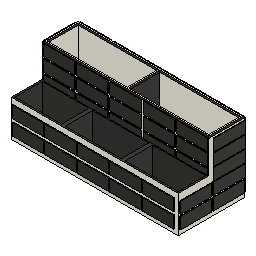
remote holder (Autodesk Fusion 360 design; units mm, degrees)
part number: 2026-07-13-07-00-43-273
Autodesk Fusion 360 part; units mm, degrees
note: some values were not read from the file. Chosen so that the rebuilt part matches the saved one: which bodies a step acts on; which face or edge a step refers to.
sketch "Sketch1" plane through (0, 0, 0) normal (0, 1, 0) x (1, 0, 0)
  line L0 (-254.9432, 107.7823) -> (245.0568, 107.7823)
  line L1 (245.0568, 107.7823) -> (245.0568, -92.2177)
  line L2 (245.0568, -92.2177) -> (-254.9432, -92.2177)
  line L3 (-254.9432, -92.2177) -> (-254.9432, 107.7823)
  line L4 (-254.9432, 0) -> (245.0568, 0)
  line L5 (0, 107.7823) -> (0, 0)
  line L6 (-100, 0) -> (-100, -92.2177)
  line L7 (80, 0) -> (80, -92.2177)
  line L8 (69.6475, -92.2177) -> (69.6475, 0)
  line L9 (-109.7986, -92.2177) -> (-109.7986, 0)
  line L10 (-10, 0) -> (-10, 107.7823)
  dimension "d1" = 500
  dimension "d2" = 200
  constraint horizontal L0
  constraint vertical L1
  constraint horizontal L2
  constraint vertical L3
  constraint coincident L3 L4.start
  constraint coincident L1 L4.end
  constraint perpendicular L1 L4
  constraint coincident L0 L5.start
  constraint coincident L5.end origin
  constraint perpendicular L4 L5
  constraint coincident L4 L6.start
  constraint coincident L2 L6.end
  constraint perpendicular L2 L6
  constraint coincident L4 L7.start
  constraint coincident L2 L7.end
  constraint perpendicular L2 L7
  constraint coincident L2 L8.start
  constraint coincident L4 L8.end
  constraint perpendicular L4 L8
  constraint coincident L2 L9.start
  constraint coincident L4 L9.end
  constraint perpendicular L4 L9
  constraint coincident L4 L10.start
  constraint coincident L0 L10.end
  constraint perpendicular L0 L10
  measures "d1" distance of L1 L3
  measures "d2" distance of L0.start L2.end
extrude "Extrude1" add sketch "Sketch1" along normal blind 100 contours L2 L3 L4 L9 | L2 L4 L6 L8 | L2 L4 L6 L9 | L1 L2 L4 L7 | L2 L4 L7 L8 makes body 1
shell "Shell2" thickness 5 removed faces 1 at (-13.4508, 100, 61.4784) on bodies 1
extrude "Extrude2" add sketch "Sketch1" along normal blind 200 contours L0 L3 L4 L10 | L0 L4 L5 L10 | L0 L1 L4 L5 bodies 1
extrude "Extrude3" add sketch "Sketch1" against normal blind 10 bodies 1
shell "Shell1" thickness 10 removed faces 1 at (-88.2765, 200, -35.9274) on bodies 1
extrude "Extrude4" add sketch "Sketch1" along normal blind 100 thin wall 1 inside contours L1 L2 L4 L7 bodies 1
extrude "Extrude5" add sketch "Sketch1" along normal blind 100 thin wall 1 inside contours L2 L4 L6 L8 | L2 L4 L7 L8 bodies 1
extrude "Extrude8" add sketch "Sketch1" along normal blind 200 contours L0 L4 L5 L10 bodies 1
extrude "Extrude9" add sketch "Sketch1" along normal blind 100 separate body contours L2 L4 L6 L9 | L2 L4 L7 L8 makes body 2 at (-100, 66.6667, 30.7392) makes body 3 at (80, 66.6667, 30.7392)
combine "Combine4" operation add target body 1 tool bodies 2 3
extrude "Extrude6" add sketch "Sketch1" along normal blind 200 thin wall 1 inside contours L0 L3 L4 L10 | L0 L4 L5 L10 bodies 1
ref_plane "WorkPlane1" through (-4.9432, 50, 92.2177) normal (0, 0, 1) x (1, 0, 0)
sketch "Sketch2" plane through (0, 0, 92.2177) normal (0, 0, 1) x (1, 0, 0)
  line L0 (-250, 83.3333) -> (-156, 83.3333)
  line L1 (-156, 83.3333) -> (-156, 48.3333)
  line L2 (-156, 48.3333) -> (-250, 48.3333)
  line L3 (-250, 48.3333) -> (-250, 83.3333)
  line L4 (-152.5, 83.3333) -> (-58.5, 83.3333)
  line L5 (-58.5, 83.3333) -> (-58.5, 48.3333)
  line L6 (-152.5, 48.3333) -> (-152.5, 83.3333)
  line L7 (-58.5, 48.3333) -> (-152.5, 48.3333)
  line L8 (-55, 83.3333) -> (39, 83.3333)
  line L9 (39, 83.3333) -> (39, 48.3333)
  line L10 (-55, 48.3333) -> (-55, 83.3333)
  line L11 (39, 48.3333) -> (-55, 48.3333)
  line L12 (42.5, 83.3333) -> (136.5, 83.3333)
  line L13 (136.5, 83.3333) -> (136.5, 48.3333)
  line L14 (42.5, 48.3333) -> (42.5, 83.3333)
  line L15 (136.5, 48.3333) -> (42.5, 48.3333)
  line L16 (140, 83.3333) -> (234, 83.3333)
  line L17 (234, 83.3333) -> (234, 48.3333)
  line L18 (140, 48.3333) -> (140, 83.3333)
  line L19 (234, 48.3333) -> (140, 48.3333)
  line L20 (-250, 38.3333) -> (-156, 38.3333)
  line L21 (-156, 38.3333) -> (-156, 3.3333)
  line L22 (-250, 3.3333) -> (-250, 38.3333)
  line L23 (-156, 3.3333) -> (-250, 3.3333)
  line L24 (-152.5, 38.3333) -> (-58.5, 38.3333)
  line L25 (-58.5, 38.3333) -> (-58.5, 3.3333)
  line L26 (-152.5, 3.3333) -> (-152.5, 38.3333)
  line L27 (-58.5, 3.3333) -> (-152.5, 3.3333)
  line L28 (-55, 38.3333) -> (39, 38.3333)
  line L29 (39, 38.3333) -> (39, 3.3333)
  line L30 (-55, 3.3333) -> (-55, 38.3333)
  line L31 (39, 3.3333) -> (-55, 3.3333)
  line L32 (42.5, 38.3333) -> (136.5, 38.3333)
  line L33 (136.5, 38.3333) -> (136.5, 3.3333)
  line L34 (42.5, 3.3333) -> (42.5, 38.3333)
  line L35 (136.5, 3.3333) -> (42.5, 3.3333)
  line L36 (140, 38.3333) -> (234, 38.3333)
  line L37 (234, 38.3333) -> (234, 3.3333)
  line L38 (140, 3.3333) -> (140, 38.3333)
  line L39 (234, 3.3333) -> (140, 3.3333)
  dimension "d25" = 94
  dimension "d28" = 390
  dimension "d29" = -45
  measures "d25" distance of L0.start L0.end
extrude "Extrude7" add sketch "Sketch2" along normal blind 3 separate body makes body 4 at (-23.6667, 26.6667, 92.2177) makes body 5 at (73.8333, 71.6667, 92.2177) makes body 6 at (-218.6667, 71.6667, 92.2177) makes body 7 at (171.3333, 71.6667, 92.2177) makes body 8 at (-121.1667, 15, 92.2177) makes body 9 at (73.8333, 26.6667, 92.2177) makes body 10 at (-23.6667, 71.6667, 92.2177) makes body 11 at (-121.1667, 60, 92.2177) makes body 12 at (171.3333, 26.6667, 92.2177) makes body 13 at (-218.6667, 26.6667, 92.2177)
copy_body "CopyPasteBodies1" bodies 7 makes body 14
move_body "Move1" bodies 14 to x (0, 0, -1) y (0, 1, 0) z (1, 0, 0) at (151.7676, 10, 222.2029)
move_body "Move2" bodies 14 to x (1, 0, 0) y (0, 1, 0) z (0, 0, 1) at (0, 0, 5)
pattern_linear "R-Pattern1" count 2 spacing 98 along (0, 0, -1) of bodies 14 makes body 15
pattern_linear "R-Pattern2" count 2 spacing 40 along (0, -1, 0) of bodies 14 makes body 16
pattern_linear "R-Pattern3" count 2 spacing 100 along (0, 0, -1) of bodies 14 16 makes body 17 at (243.9853, 81.6667, -44.1304) makes body 18 at (243.9853, 41.6667, -44.1304)
pattern_linear "R-Pattern4" count 3 spacing 52.5 along (0, 1, 0) of bodies 17 makes body 19 at (243.9853, 134.1667, -44.1304) makes body 20 at (243.9853, 186.6667, -44.1304)
move_body "Move3" bodies 19 20 to x (1, 0, 0) y (0, 1, 0) z (0, 0, 1) at (0, 0, 5)
move_body "Move4" bodies 19 20 to x (1, 0, 0) y (0, 1, 0) z (0, 0, 1) at (0, 0, -5)
move_body "Move5" bodies 16 14 20 15 19 18 17 to x (1, 0, 0) y (0, 1, 0) z (0, 0, 1) at (0, -15, 0)
move_body "Move6" bodies 19 to x (1, 0, 0) y (0, 1, 0) z (0, 0, 1) at (0, -15, 0)
move_body "Move7" bodies 20 to x (1, 0, 0) y (0, 1, 0) z (0, 0, 1) at (0, -30, 0)
copy_body "CopyPasteBodies2" bodies 20 makes body 21
move_body "Move8" bodies 21 to x (1, 0, 0) y (0, 1, 0) z (0, 0, 1) at (0, 38, 0)
move_body "Move9" bodies 18 to x (0, 0, -1) y (0, 1, 0) z (1, 0, 0) at (256.7823, -1, 137.1882)
pattern_linear "R-Pattern5" count 5 spacing 40 along (0, 1, 0) count 5 spacing 100 along (-1, 0, 0) of bodies 18 makes body 22 at (212.652, 65.6667, -106.7971) makes body 23 at (212.652, 105.6667, -106.7971) makes body 24 at (212.652, 145.6667, -106.7971) makes body 25 at (212.652, 185.6667, -106.7971) makes body 26 at (112.652, 25.6667, -106.7971) makes body 27 at (112.652, 65.6667, -106.7971) makes body 28 at (112.652, 105.6667, -106.7971) makes body 29 at (112.652, 145.6667, -106.7971) makes body 30 at (112.652, 185.6667, -106.7971) makes body 31 at (12.652, 25.6667, -106.7971) makes body 32 at (12.652, 65.6667, -106.7971) makes body 33 at (12.652, 105.6667, -106.7971) makes body 34 at (12.652, 145.6667, -106.7971) makes body 35 at (12.652, 185.6667, -106.7971) makes body 36 at (-87.348, 25.6667, -106.7971) makes body 37 at (-87.348, 65.6667, -106.7971) makes body 38 at (-87.348, 105.6667, -106.7971) makes body 39 at (-87.348, 145.6667, -106.7971) makes body 40 at (-87.348, 185.6667, -106.7971) makes body 41 at (-187.348, 25.6667, -106.7971) makes body 42 at (-187.348, 65.6667, -106.7971) makes body 43 at (-187.348, 105.6667, -106.7971) makes body 44 at (-187.348, 145.6667, -106.7971) makes body 45 at (-187.348, 185.6667, -106.7971)
copy_body "CopyPasteBodies3" bodies 16 makes body 46
move_body "Move10" bodies 46 to x (1, 0, 0) y (0, 1, 0) z (0, 0, 1) at (0, 0, -98)
move_body "Move11" bodies 45 to x (0, 0, -1) y (0, 1, 0) z (1, 0, 0) at (-147.4048, 0, -256.9989)
pattern_linear "R-Pattern6" count 5 spacing 40 along (0, -1, 0) of bodies 45 makes body 47 at (-254.2018, 145.6667, -69.6508) makes body 48 at (-254.2018, 105.6667, -69.6508) makes body 49 at (-254.2018, 65.6667, -69.6508) makes body 50 at (-254.2018, 25.6667, -69.6508)
copy_body "CopyPasteBodies4" bodies 49 50 makes body 51 makes body 52
move_body "Move12" bodies 51 52 to x (1, 0, 0) y (0, 1, 0) z (0, 0, 1) at (0, 1, 98)
copy_body "CopyPasteBodies5" bodies 44 makes body 53
move_body "Move13" bodies 53 to x (1, 0, 0) y (0, 1, 0) z (0, 0, 1) at (0, 40, 0)
move_body "Move14" bodies 25 to x (1, 0, 0) y (0, 1, 0) z (0, 0, 1) at (0, 0, 109)
pattern_linear "R-Pattern7" count 5 spacing 100 along (-1, 0, 0) count 5 spacing 40 along (0, -1, 0) of bodies 25 makes body 54 at (112.652, 185.6667, 2.2029) makes body 55 at (12.652, 185.6667, 2.2029) makes body 56 at (-87.348, 185.6667, 2.2029) makes body 57 at (-187.348, 185.6667, 2.2029) makes body 58 at (212.652, 145.6667, 2.2029) makes body 59 at (112.652, 145.6667, 2.2029) makes body 60 at (12.652, 145.6667, 2.2029) makes body 61 at (-87.348, 145.6667, 2.2029) makes body 62 at (-187.348, 145.6667, 2.2029) makes body 63 at (212.652, 105.6667, 2.2029) makes body 64 at (112.652, 105.6667, 2.2029) makes body 65 at (12.652, 105.6667, 2.2029) makes body 66 at (-87.348, 105.6667, 2.2029) makes body 67 at (-187.348, 105.6667, 2.2029) makes body 68 at (212.652, 65.6667, 2.2029) makes body 69 at (112.652, 65.6667, 2.2029) makes body 70 at (12.652, 65.6667, 2.2029) makes body 71 at (-87.348, 65.6667, 2.2029) makes body 72 at (-187.348, 65.6667, 2.2029) makes body 73 at (212.652, 25.6667, 2.2029) makes body 74 at (112.652, 25.6667, 2.2029) makes body 75 at (12.652, 25.6667, 2.2029) makes body 76 at (-87.348, 25.6667, 2.2029) makes body 77 at (-187.348, 25.6667, 2.2029)
move_body "Move15" bodies 24 to x (1, 0, 0) y (0, 1, 0) z (0, 0, 1) at (0, 40, 0)
copy_body "CopyPasteBodies6" bodies 57 makes body 78
move_body "Move16" bodies 78 to x (1, 0, 0) y (0, 1, 0) z (0, 0, 1) at (0, -40, 0)
copy_body "CopyPasteBodies7" bodies 24 makes body 79
move_body "Move17" bodies 79 to x (1, 0, 0) y (0, 1, 0) z (0, 0, 1) at (0, -40, 0)
combine "Combine3" operation add target body 1 tool bodies 4 5 6 7 9 8 10 11 12 13 14 15 16 17 18 19 20 21 22 23 24 25 26 27 28 29 30 31 32 33 35 34 36 37 38 40 39 41 42 43 44 45 46 47 48 49 51 50 52 53
chamfer "Chamfer1" distance 3 angle 45 1 faces at (-3.2955, 200, -3.3333) on bodies 1
fillet "Fillet2" radius 0.1 4 edges at (-3, 200, -53.8912) (-1.5, 198.5, -8.5) (0, 197, -53.8912) (-1.5, 198.5, -99.2823) on bodies 1
combine "Combine5" operation add target body 1 tool bodies 60 55 56 64 65 61 58 63 59 57 67 54 62 66 68 69 70 72 71 73 74 75 76 77
combine "Combine6" operation add target body 1 tool bodies 78
combine "Combine7" operation add target body 1 tool bodies 79
scale "Scale1" factor 0.25 about (-99, 100, 5) bodies 1
move_body "Move18" bodies 1 to x (1, 0, 0) y (0, 1, 0) z (0, 0, 1) at (75.4858, -72.5, -1.8044)
named bodies: "main"
